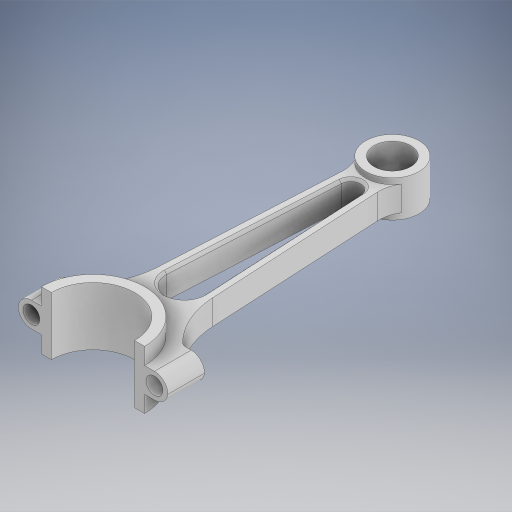
# Autodesk Inventor part: LE-2.1
Saved by Autodesk Inventor 2024 (Build 280153000, 153)
## iProperties
Created: 2024-02-01
Part Number: LE-2.1
Material: Generic
Document SubType Name: Modeling
Designer: Alex
Density: 1 g/cm^3
Appearance: Default
Author: Alex
Autodesk Inventor part; units mm, degrees
ref_plane "YZ Plane" through (0, 0, 0) normal (1, 0, 0) x (0, 1, 0)
ref_plane "XZ Plane" through (0, 0, 0) normal (0, 1, 0) x (-1, 0, 0)
ref_plane "XY Plane" through (0, 0, 0) normal (0, 0, 1) x (1, 0, 0)
sketch "Sketch1" plane through (0, 0, 0) normal (0, 1, 0) x (-1, 0, 0)
  arc A0 (-31, 0) -> (31, 0) centre (0, 0) ccw
  arc A1 (-25, 0) -> (25, 0) centre (0, 0) ccw
  line L0 (25, 0) -> (31, 0)
  line L1 (0, 31) -> (0, -180) construction
  line L2 (-25, 0) -> (-31, 0)
  circle A2 centre (0, -180) radius 11
  circle A3 centre (0, -180) radius 16
  line L3 (0, -180) -> (36.7179, -180) construction
  line L4 (0, -55) -> (36.7179, -55) construction
  line L5 (0, -155) -> (36.7179, -155) construction
  arc A4 (-5.9918, -155.314) -> (6, -155) centre (0, -155) ccw
  line L6 (-11.2182, -55.5879) -> (-5.9918, -155.314)
  line L7 (-16.2113, -55.8496) -> (-10.7437, -160.1781)
  arc A5 (11.2182, -55.5879) -> (-11.2182, -55.5879) centre (0, -55) ccw
  line L8 (11.2182, -55.5879) -> (5.9918, -155.314)
  arc A6 (-13.6517, -171.6555) -> (-10.7437, -160.1781) centre (-30.7163, -161.2248) ccw
  line L9 (0, -55) -> (-28, -55) construction
  line L10 (0, -55) -> (-66.1428, -58.4664) construction
  circle A7 centre (-66.1428, -58.4664) radius 50 construction
  line L11 (-31, 0) -> (-37, 0)
  line L12 (31, 0) -> (37, 0)
  line L13 (-37, 0) -> (-37, -22)
  line L14 (-37, -22) -> (-33.9735, -22)
  arc A8 (-30.3991, -23.5037) -> (-33.9735, -22) centre (-33.9735, -27) ccw
  arc A9 (-16.2113, -55.8496) -> (-30.3991, -23.5037) centre (-66.1428, -58.4664) ccw
  line L15 (16.2113, -55.8496) -> (10.7437, -160.1781)
  arc A10 (10.7437, -160.1781) -> (13.6517, -171.6555) centre (30.7163, -161.2248) ccw
  line L16 (37, 0) -> (37, -22)
  line L17 (37, -22) -> (33.9735, -22)
  arc A11 (33.9735, -22) -> (30.3991, -23.5037) centre (33.9735, -27) ccw
  arc A12 (30.3991, -23.5037) -> (16.2113, -55.8496) centre (66.1428, -58.4664) ccw
  point P0 (0, -13.7481)
  point P1 (13.6517, -171.6555)
  dimension "d10" = 32
  dimension "d20" = 100
  dimension "d0" = 62
  dimension "d1" = 50
  dimension "d6" = 0
  dimension "d7" = 31
  dimension "d9" = 22
  dimension "d11" = 125
  dimension "d12" = 100
  dimension "d13" = 12
  dimension "d15" = 3
  dimension "d16" = 5
  dimension "d17" = 180
  dimension "d18" = 40
  dimension "d19" = 3
  dimension "d22" = 74
  dimension "d23" = 22
  dimension "d24" = 10
  constraints: 37 end point, 20 point on circle, 14 symmetric about line, 11 centre point, 5 point on line, 4 coincident, 4 horizontal, 4 tangent, 3 parallel, 2 vertical, 1 perpendicular, 13 other
  measures "d0" diameter of A0
  measures "d1" diameter of A1
  measures "d6" distance from line of point (0, 0) L2
  measures "d7" distance from line of L1.start L2
  measures "d9" diameter of A2
  measures "d11" distance between parallel lines of L3 L4
  measures "d12" distance between parallel lines of L4 L5
  measures "d13" diameter of A4
  measures "d15" angle of L1 L6
  measures "d16" distance between parallel lines of L6 L7
  measures "d17" distance of point (0, 0) L1.end
  measures "d18" diameter of A6
  measures "d19" angle of L9 L10
  measures "d22" distance of L11.end L12.end
  measures "d23" distance of L11.end L13.end
  measures "d24" diameter of A8
extrude "Extrusion1" add sketch "Sketch1" along normal mid plane 35 contours L2 A1 L0 A0
extrude "Extrusion2" add sketch "Sketch1" along normal mid plane 15 contours A0 L12 L16 L17 A11 A12 L15 A10 A3 A6 L7 A9 A8 L14 L13 L11
extrude "Extrusion3" add sketch "Sketch1" along normal mid plane 22 contours A3
sketch "Sketch2" plane through (25, 17.5, 0) normal (0, 0, 1) x (1, 0, 0)
  line L0 (6, -35) -> (6, -25) construction
  line L1 (12, -25) -> (6, -25) construction
  line L2 (12, -25) -> (12, -10) projected
  line L3 (6, -10) -> (12, -10) construction
  line L4 (6, -10) -> (6, 0) construction
  line L5 (0, 0) -> (6, 0) construction
  line L6 (0, -35) -> (0, 0) construction
  line L7 (6, -35) -> (0, -35) construction
  line L8 (-55.3991, -25) -> (-55.3991, -10) construction
  line L9 (-50, -35) -> (-50, 0) construction
  line L10 (-56, 0) -> (-50, 0) construction
  line L11 (-56, 0) -> (-56, -10) construction
  line L12 (-62, -10) -> (-56, -10) construction
  line L13 (-62, -25) -> (-62, -10) construction
  line L14 (-56, -25) -> (-62, -25) construction
  line L15 (-56, -25) -> (-56, -35) construction
  line L16 (-50, -35) -> (-56, -35) construction
  line L17 (0, -35) -> (0, 0) construction
  line L18 (-50, 0) -> (0, 0) construction
  line L19 (-50, -35) -> (-50, 0) construction
  line L20 (0, -35) -> (-50, -35) construction
  line L21 (-25, 0) -> (-25, -35) construction
  circle A0 centre (12, -17.5) radius 5
  line L22 (12, -10) -> (8.9735, -10) projected
  line L23 (12, -10) -> (20, -10)
  line L24 (-25, -17.5) -> (12, -17.5) construction
  line L25 (12, -25) -> (12, -10) construction
  line L26 (12, -25) -> (20, -25)
  line L27 (20, -10) -> (20, -25)
  point P0 (12, -12.5)
  point P1 (12, -22.5)
  dimension "d31" = 10
  dimension "d32" = 8
  constraints: 10 end point, 3 midpoint, 1 centre point, 1 perpendicular, 1 point on line, 1 symmetric about line, 1 vertical
  measures "d31" diameter of A0
  measures "d32" distance of L2.end L23.end
extrude "Extrusion4" add sketch "Sketch2" against normal blind 22 contours L2 A0 L23 L27 L26
extrude "Extrusion5" cut sketch "Sketch2" against normal through all contours A0 L2 picked at (10.8948, -16.2525)
fillet "Fillet1" radius 8 2 edges at (45, 7.5, -11) (45, -7.5, -11)
mirror "Mirror1" about plane through (0, 0, 0) normal (1, 0, 0) of "Fillet1", "Extrusion4", "Extrusion5"
chamfer "Chamfer1" distance 1.5 angle 45 4 edges at (-8.605, 7.5, -105.451) (0, 7.5, -161) (8.605, 7.5, -105.451) (0, 7.5, -43.7664)
ref_plane "Work Plane1" through (0, 0, 0) normal (1, 0, 0) x (0, 1, 0)
body "Solid1"
